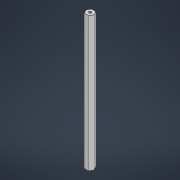
# Autodesk Inventor part: Spacer_M3-Hex7-L130
Saved by Autodesk Inventor 2022.4 (Build 264492010, 492A)
## iProperties
Created: 2023-06-19
Part Number: Spacer_M3-Hex7-L130
Material: 一般
Document SubType Name: Modeling
Designer: 22-ayato
Density: 1 g/cm^3
Appearance: 既定
Author: 22-ayato
Autodesk Inventor part; units mm, degrees
ref_plane "YZ Plane" through (0, 0, 0) normal (1, 0, 0) x (0, 1, 0)
ref_plane "XZ Plane" through (0, 0, 0) normal (0, 1, 0) x (-1, 0, 0)
ref_plane "XY Plane" through (0, 0, 0) normal (0, 0, 1) x (1, 0, 0)
sketch "スケッチ1" plane through (0, 0, 0) normal (0, 1, 0) x (-1, 0, 0)
  line L0 (2.0207, 3.5) -> (4.0415, 0)
  line L1 (4.0415, 0) -> (2.0207, -3.5)
  line L2 (2.0207, -3.5) -> (-2.0207, -3.5)
  line L3 (-2.0207, -3.5) -> (-4.0415, 0)
  line L4 (-4.0415, 0) -> (-2.0207, 3.5)
  line L5 (-2.0207, 3.5) -> (2.0207, 3.5)
  point P0 (0, 0)
  point P1 (0, 0)
  dimension "d0" = 7
  constraints: 12 end point, 1 coincident, 1 horizontal alignment, 13 other
  measures "d0" distance between parallel lines of L2 L5
extrude "押し出し1" add sketch "スケッチ1" along normal mid plane 130
sketch "スケッチ2" plane through (0, 65, 0) normal (0, 1, 0) x (1, 0, 0)
  point P0 (0, 0)
  point P1 (0, 0)
  constraints: 1 coincident
hole "穴1" at (0, 65, 0) direction (0, -1, 0) diameter 2.459 end through all thread size "M3x0.5" class "6H" standard "ISO Metric profile"
chamfer "面取り1" distance 0.2 angle 45 2 edges at (0, 65, -1.2295) (0, -65, -1.2295)
chamfer "面取り2" distance 0.2 angle 45 12 edges at (0, 65, 3.5) (-3.0311, 65, 1.75) (-3.0311, 65, -1.75) (0, 65, -3.5) (3.0311, 65, -1.75) (3.0311, 65, 1.75) (3.0311, -65, 1.75) (3.0311, -65, -1.75) (0, -65, 3.5) (-3.0311, -65, 1.75) (-3.0311, -65, -1.75) (0, -65, -3.5)
